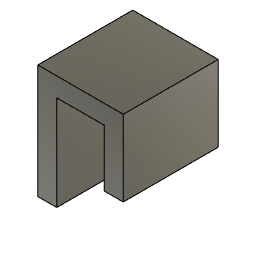
Wire_clip (Autodesk Fusion 360 design; units mm, degrees)
Autodesk Fusion 360 part; units mm, degrees
sketch "Sketch1" plane through (0, 0, 0) normal (0, 0, 1) x (1, 0, 0)
  line L0 (0, 0) -> (2, 0)
  line L1 (2, 0) -> (2, 10)
  line L2 (2, 10) -> (0, 10)
  line L3 (0, 10) -> (0, 0)
  dimension "d4" = 10
  dimension "d5" = 2
  constraint horizontal L0
  constraint vertical L1
  constraint horizontal L2
  constraint vertical L3
  constraint coincident L0.start L3.end
  measures "d4" distance of L0.end L1.end
  measures "d5" distance of L1.end L2.end
extrude "Extrude1" add sketch "Sketch1" along normal blind 12
sketch "Sketch2" plane through (2, 0, 0) normal (1, 0, 0) x (0, 1, 0)
  line L0 (0, 0) -> (10, 0)
  line L1 (10, 0) -> (10, 12)
  line L2 (10, 12) -> (0, 12)
  line L3 (0, 12) -> (0, 0)
  line L4 (0, 12) -> (10, 12)
  line L5 (10, 12) -> (10, 10)
  line L6 (10, 10) -> (0, 10)
  line L7 (0, 10) -> (0, 12)
  dimension "d8" = 2
  constraint horizontal L4
  constraint vertical L5
  constraint horizontal L6
  constraint vertical L7
  constraint coincident L2.end L3.start
  constraint coincident L1.end L5
  measures "d8" distance of L2.end L6.end
extrude "Extrude2" add sketch "Sketch2" along normal blind 7 contours L1 L2 L3 L4 L5 L6 L7
sketch "Sketch3" plane through (0, 0, 10) normal (0, 0, -1) x (1, 0, 0)
  line L0 (2, 0) -> (2, -10)
  line L1 (2, -10) -> (9, -10)
  line L2 (9, -10) -> (9, 0)
  line L3 (9, 0) -> (2, 0)
  line L4 (9, -10) -> (7, -10)
  line L5 (7, -10) -> (7, 0)
  line L6 (7, 0) -> (9, 0)
  line L7 (9, 0) -> (9, -10)
  dimension "d11" = 2
  constraint horizontal L4
  constraint vertical L5
  constraint horizontal L6
  constraint vertical L7
  constraint coincident L1.end L2.start
  measures "d11" distance of L1.end L4.end
extrude "Extrude3" add sketch "Sketch3" along normal blind 6 contours L1 L2 L3 L4 L5 L6 L7
equation "width = 10 mm"
equation "length = 2 mm"
equation "height = 12 mm"
equation "d4 = width"
equation "d5 = length"
equation "d6 = height"
